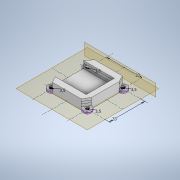
# Autodesk Inventor part: Electro_lora
Saved by Autodesk Inventor 2020 (Build 240168000, 168)
## iProperties
Created: 2020-09-03
Part Number: Electro_lora
Material: Generisch
Document SubType Name: Modeling
Designer: sp
Density: 1 g/cm^3
Appearance: Vorgabe
Author: sp
## iProperties of the stored document _3D-Druck.ipt
Created: 2022-05-23
Part Number: _3D-Druck
Material: Generisch
Document SubType Name: Modeling
Designer: sp
Density: 1 g/cm^3
Appearance: Vorgabe
Author: sp
Autodesk Inventor part; units mm, degrees
ref_plane "YZ Plane" through (0, 0, 0) normal (1, 0, 0) x (0, 1, 0)
sketch "Skizze1" plane through (0, 0, 0) normal (0, 1, 0) x (-1, 0, 0)
  circle A0 centre (0, 0) radius 30
  circle A1 centre (0, 0) radius 27
  dimension "d0" = 60
  dimension "d1" = 54
  constraints: 2 centre point, 2 coincident
  measures "d0" diameter of A0
  measures "d1" diameter of A1
extrude "Extrusion1" add sketch "Skizze1" along normal mid plane 10
sketch "Skizze5" plane through (0, 0, 0) normal (0, 1, 0) x (-1, 0, 0)
  line L0 (12.75, -14.75) -> (-12.75, -14.75)
  line L1 (-12.75, -14.75) -> (-12.75, 14.75)
  line L2 (-12.75, 14.75) -> (12.75, 14.75)
  line L3 (12.75, 14.75) -> (12.75, -14.75)
  line L4 (49.4097, 0) -> (-52.5504, 0) construction
  line L5 (0, -53.7913) -> (0, 68.1535) construction
  line L6 (-16.75, -18.75) -> (16.75, -18.75)
  line L7 (16.75, -18.75) -> (16.75, 18.75)
  line L8 (16.75, 18.75) -> (-16.75, 18.75)
  line L9 (-16.75, 18.75) -> (-16.75, -18.75)
  point P0 (0, 0)
  dimension "d33" = 29.5
  dimension "d34" = 25.5
  dimension "d35" = 4
  constraints: 20 end point, 4 parallel, 2 horizontal, 2 perpendicular, 2 point on line, 1 vertical, 5 other
  measures "d33" distance of L0.end L1.end
  measures "d34" distance of L0.start L0.end
  measures "d35" distance between parallel lines of L0 L6
extrude "Extrusion5" add sketch "Skizze5" along normal mid plane 2.5 contours L0 L1 L2 L3 | L9 L8 L7 L6
ref_plane "Arbeitsebene1" through (0, 0, 0) normal (0, 1, 0) x (-1, 0, 0)
chamfer "Fase1" distance 1 angle 45 2 edges at (30, 5, 0) (30, -5, 0)
sketch "Skizze2" plane through (0, 0, 0) normal (0, 1, 0) x (-1, 0, 0)
  line L0 (0, 42.2301) -> (0, -36.7007) construction
  line L1 (32.6355, 0) -> (-32.6355, 0) construction
  line L2 (16.5, 34.419) -> (16.5, -40.3324) construction
  line L3 (-16.5, 35.4304) -> (-16.5, -34.8157) construction
  line L4 (23.5881, 16.5) -> (-32.0387, 16.5) construction
  line L5 (23.5881, -16.5) -> (-39.8541, -16.5) construction
  circle A0 centre (16.5, -16.5) radius 1.75
  circle A1 centre (16.5, 16.5) radius 1.75
  circle A2 centre (-16.5, 16.5) radius 1.75
  circle A3 centre (-16.5, -16.5) radius 1.75
  circle A4 centre (-16.5, 16.5) radius 3.6749
  circle A5 centre (-16.5, -16.5) radius 3.7161
  circle A6 centre (16.5, -16.5) radius 3.7
  circle A7 centre (16.5, 16.5) radius 3.6747
  point P0 (0, 0)
  dimension "d8" = 33
  dimension "d9" = 33
  dimension "d10" = 3.5
  dimension "d11" = 3.5
  dimension "d12" = 3.5
  dimension "d13" = 3.5
  constraints: 12 end point, 9 point on line, 8 centre point, 4 coincident, 3 horizontal, 3 vertical, 1 midpoint, 2 other
  measures "d8" distance between parallel lines of L3 L2
  measures "d9" distance between parallel lines of L4 L5
  measures "d10" diameter of A0
  measures "d11" diameter of A1
  measures "d12" diameter of A2
  measures "d13" diameter of A3
extrude "Extrusion2" add sketch "Skizze2" along normal mid plane 2.5
ref_plane "Arbeitsebene2" through (0, 0, -30.5) normal (0, 0, 1) x (1, 0, 0)
sketch "Skizze4" plane through (0, 0, -30.5) normal (0, 0, 1) x (1, 0, 0)
  circle A0 centre (0, 0) radius 1.75
  dimension "d27" = 3.5
  constraints: 1 centre point, 1 coincident
  measures "d27" diameter of A0
extrude "Extrusion4" cut sketch "Skizze4" along normal blind 5
pattern_circular "Runde Anordnung1" count 3 over 360 about axis through (0, -10, 0) along (0, 1, 0) of "Extrusion4"
extrude "Extrusion6" cut sketch "Skizze2" against normal mid plane 3 contours A0 | A1 | A2 | A3
sketch "Skizze9" plane through (0, 1.25, 0) normal (0, 1, 0) x (1, 0, 0)
  line L0 (-69.7696, 0) -> (96.0942, 0) construction
  line L1 (0, -81.4667) -> (0, 124.1465) construction
  line L2 (-12, -13) -> (12, -13)
  line L3 (12, -13) -> (12, 13)
  line L4 (12, 13) -> (-12, 13)
  line L5 (-12, 13) -> (-12, -13)
  line L6 (-16.75, 12.8084) -> (-16.75, -12.8338) projected
  line L7 (-16.75, -12.8338) -> (-16.75, 12.8084)
  line L8 (-16.75, 12.8084) -> (-12, 18.75)
  line L9 (-13.5627, 18.75) -> (13.5425, 18.75) projected
  arc A0 (18.6215, 19.551) -> (13.5425, 18.75) centre (16.5, 16.5) ccw projected
  line L10 (-12, 18.75) -> (13.5425, 18.75)
  line L11 (13.5425, 18.75) -> (16.75, 12.7361)
  line L12 (16.75, -12.8336) -> (16.75, 12.7924) projected
  line L13 (16.75, 12.7361) -> (16.75, -12.8336)
  line L14 (16.75, -12.8336) -> (13.1623, -18.75)
  line L15 (-13.5947, -18.75) -> (13.5944, -18.75) projected
  arc A1 (-18.8927, -19.289) -> (-13.5947, -18.75) centre (-16.5, -16.5) ccw projected
  line L16 (13.1623, -18.75) -> (-13.5947, -18.75)
  line L17 (-13.5947, -18.75) -> (-16.75, -12.8338)
  line L18 (-12, 13) -> (-16.5968, 13)
  line L19 (-12, -13) -> (-16.6614, -13)
  point P0 (0, 0)
  dimension "d46" = 26
  dimension "d47" = 24
  constraints: 32 end point, 6 point on line, 5 horizontal, 4 parallel, 2 vertical, 1 collinear, 1 perpendicular, 2 other
  measures "d46" distance of L4.end L2.start
  measures "d47" distance of L3.end L4.end
extrude "Extrusion10" add sketch "Skizze9" along normal blind 2.5 contours L2 L3 L4 L18 L8 L9 L11 L12 L14 L15 L17 L19
sketch "Skizze10" plane through (0, 3.75, 0) normal (0, 1, 0) x (1, 0, 0)
  line L0 (-13, -15) -> (13, -15)
  line L1 (13, -15) -> (13, 15)
  line L2 (13, 15) -> (-13, 15)
  line L3 (-13, 15) -> (-13, -15)
  line L4 (0, -23.0376) -> (0, 31.543) construction
  line L5 (-22.6834, 0) -> (18.5133, 0) construction
  arc A0 (18.6215, 19.551) -> (13.5425, 18.75) centre (16.5, 16.5) ccw projected
  line L6 (-12, 18.75) -> (13.5425, 18.75)
  line L7 (13.5944, -18.75) -> (-13.5947, -18.75) projected
  line L8 (-13.5947, -18.75) -> (13.5944, -18.75)
  line L9 (-13, 15) -> (-12, 18.75)
  arc A1 (-18.8927, -19.289) -> (-13.5947, -18.75) centre (-16.5, -16.5) ccw projected
  line L10 (-13, -15) -> (-13.5947, -18.75)
  line L11 (16.75, 12.7924) -> (16.75, -12.8336) projected
  arc A2 (16.75, 12.7924) -> (19.551, 18.6215) centre (16.5, 16.5) ccw projected
  line L12 (16.75, -12.8336) -> (16.75, 12.7924)
  line L13 (16.75, 12.7361) -> (13.5425, 18.75) projected
  line L14 (16.75, 12.7924) -> (13.5425, 18.75)
  line L15 (16.75, -12.8336) -> (15.2979, -15.2282) projected
  line L16 (16.75, -12.8336) -> (13.1918, -18.75)
  point P0 (0, 0)
  dimension "d50" = 30
  dimension "d51" = 26
  constraints: 26 end point, 4 horizontal, 3 point on line, 2 parallel, 2 vertical, 1 perpendicular, 2 other
  measures "d50" distance between parallel lines of L2 L0
  measures "d51" distance of L1.end L2.end
extrude "Extrusion11" add sketch "Skizze10" along normal blind 2 contours L0 L1 L2 L9 L6 L13 L11 L16 L7 L10
sketch "Skizze11" plane through (0, 5.75, 0) normal (0, 1, 0) x (1, 0, 0)
  line L0 (12, 13) -> (-16.5968, 13) projected
  line L1 (-16.6614, -13) -> (-13.5947, -18.75) projected
  line L2 (12, 13) -> (-16.6614, 13)
  line L3 (-16.6614, 13) -> (-16.6614, -13)
  line L4 (-16.6614, -13) -> (12, -13)
  line L5 (12, -13) -> (12, 13)
  line L6 (13.5425, 18.75) -> (-12, 18.75) projected
  line L7 (-12, 18.75) -> (13.5425, 18.75)
  arc A0 (16.75, 12.7924) -> (19.551, 18.6215) centre (16.5, 16.5) ccw projected
  line L8 (13.5425, 18.75) -> (16.75, 12.7924)
  line L9 (16.75, 12.7924) -> (16.75, -12.8336) projected
  line L10 (16.75, 12.7924) -> (16.75, -12.8336)
  line L11 (13.1623, -18.75) -> (13.5944, -18.75) projected
  line L12 (16.75, -12.8336) -> (13.1623, -18.75)
  line L13 (13.1623, -18.75) -> (-13.5947, -18.75)
  line L14 (-16.75, 12.8084) -> (-16.75, -12.8338) projected
  line L15 (-13.5947, -18.75) -> (-16.75, -12.8338)
  line L16 (-16.6614, 13) -> (-12, 18.75)
  point P0 (0, 0)
  constraints: 22 end point, 3 parallel, 2 horizontal, 1 collinear, 1 perpendicular
extrude "Extrusion12" add sketch "Skizze11" along normal blind 2 contours L0 L2 L16 L6 L8 L9 L12 L13 L1 L4 L5
sketch "Skizze12" plane through (0, 5, 0) normal (0, 1, 0) x (1, 0, 0)
  circle A0 centre (0, 0) radius 27
  circle A1 centre (0, 0) radius 31.5802
  constraints: 2 centre point, 2 coincident
extrude "Extrusion13" cut sketch "Skizze12" against normal blind 10
